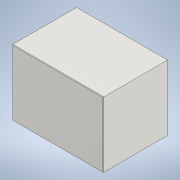
# Autodesk Inventor part: Caixa
Saved by Autodesk Inventor 2022 (Build 260153000, 153)
## iProperties
Created: 2021-09-17
Part Number: Caixa
Material: Genérico
Document SubType Name: Modeling
Designer: rubia
Density: 1 g/cm^3
Appearance: Aço
Author: rubia
Autodesk Inventor part; units mm, degrees
ref_plane "YZ Plane" through (0, 0, 0) normal (1, 0, 0) x (0, 1, 0)
ref_plane "XZ Plane" through (0, 0, 0) normal (0, 1, 0) x (-1, 0, 0)
ref_plane "XY Plane" through (0, 0, 0) normal (0, 0, 1) x (1, 0, 0)
sketch "Esboço11" plane through (0, 0, 0) normal (0, 0, 1) x (1, 0, 0)
  line L0 (0, 0) -> (354, 0)
  line L1 (354, 0) -> (354, 254)
  line L2 (354, 254) -> (0, 254)
  line L3 (0, 254) -> (0, 0)
  line L4 (2, 252) -> (352, 252)
  line L5 (352, 252) -> (352, 2)
  line L6 (352, 2) -> (2, 2)
  line L7 (2, 2) -> (2, 252)
  dimension "d14" = 354
  dimension "d15" = 254
  dimension "d16" = 2
  dimension "d17" = 2
  dimension "d18" = 2
  dimension "d19" = 2
  constraints: 16 end point, 4 parallel, 2 horizontal, 2 perpendicular
  measures "d14" distance of L2.end L1.end
  measures "d15" distance of L1.end L0.end
  measures "d16" distance between parallel lines of L1 L5
  measures "d17" distance between parallel lines of L2 L4
  measures "d18" distance between parallel lines of L3 L7
  measures "d19" distance between parallel lines of L0 L6
extrude "Extrusão3" add sketch "Esboço11" along normal blind 250
sketch "Esboço12" plane through (0, 0, 250) normal (0, 0, 1) x (1, 0, 0)
  line L0 (2, 2) -> (2, 252) projected
  line L1 (352, 2) -> (2, 2) projected
  line L2 (2, 252) -> (352, 252)
  line L3 (352, 252) -> (352, 2)
  line L4 (352, 2) -> (2, 2)
  line L5 (2, 2) -> (2, 252)
  point P0 (0, 0)
  constraints: 8 end point, 2 parallel, 1 horizontal, 1 perpendicular
extrude "Extrusão4" add sketch "Esboço12" against normal blind 2
fillet "Arredondamento1" radius 2 4 edges at (177, 254, 250) (177, 2, 248) (354, 127, 250) (0, 127, 250)
